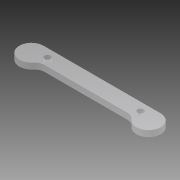
# Autodesk Inventor part: plastic_part_53
Saved by Autodesk Inventor 2013 (Build 170138000, 138)
## iProperties
Shininess: 20.0
Created: 2014-03-15
Part Number: plastic_part_53
Document SubType Name: Modeling
Designer: Noa Izumi
Material: Default
Density: 1 g/cm^3
Density: 0.0
Volumn: 0.0
Area: 0.0
PropertySet Name: Model Information
Control State: 0
Master: False
Checked Out: False
Author: Noa Izumi
Autodesk Inventor part; units mm, degrees
ref_plane "YZ Plane" through (0, 0, 0) normal (1, 0, 0) x (0, 1, 0)
ref_plane "XZ Plane" through (0, 0, 0) normal (0, 1, 0) x (-1, 0, 0)
ref_plane "XY Plane" through (0, 0, 0) normal (0, 0, 1) x (1, 0, 0)
sketch "Sketch1" plane through (0, 0, 0) normal (0, 0, 1) x (1, 0, 0)
  line L0 (0, 0) -> (58, 0)
  line L1 (58, 0) -> (58, 8)
  line L2 (58, 8) -> (0, 8)
  line L3 (0, 8) -> (0, 0)
  circle A0 centre (0, 2) radius 6
  circle A1 centre (58, 2) radius 6
  dimension "d88" = 12
  dimension "d0" = 58
  dimension "d1" = 8
  constraints: 8 end point, 2 parallel, 2 point on line, 2 vertical alignment, 1 horizontal, 1 perpendicular, 4 other
  measures "d0" distance of L0.start L0.end
  measures "d1" distance of L2.end L0.start
extrude "Extrusion1" add sketch "Sketch1" along normal blind 3
fillet "圓角5" radius 5 2 edges at (5.6569, 0, 1.5) (52.3431, 0, 1.5)
sketch "草圖9" plane through (0, 0, 3) normal (0, 0, 1) x (1, 0, 0)
  line L0 (0, 8) -> (58, 8) projected
  arc A0 (0, 8) -> (4.6283, -1.8182) centre (0, 2) ccw projected
  point P0 (0, 0)
  point P1 (6, 4)
  point P2 (52, 4)
  dimension "d90" = 4
  dimension "d91" = 46
  dimension "d92" = 6
  measures "d90" distance from line of point (6, 4) L0
  measures "d91" distance of point (52, 4) point (6, 4)
  measures "d92" horizontal distance of A0.centre point (6, 4)
hole "孔5" at (6, 4, 3) at (52, 4, 3) direction (0, 0, -1) diameter 3 end through all
